Autodesk Inventor part; units mm, degrees
note: some values were not read from the file. Chosen so that the rebuilt part matches the saved one: direction of "Hole2".
(part 17 of 20)
  spline S21 degree 3 poles (10.251041, -15.718972) (10.254521, -15.717406) (10.261436, -15.714294) (10.271248, -15.708633) (10.280531, -15.702321) (10.289255, -15.69531) (10.297429, -15.687643) (10.305055, -15.67934) (10.312135, -15.670426) (10.318671, -15.660926) (10.324667, -15.650864) (10.330124, -15.640264) (10.335046, -15.629149) (10.339434, -15.617543) (10.343295, -15.60547) (10.346618, -15.592951) (10.349454, -15.580017) (10.350882, -15.571212) (10.351603, -15.566761) knots 0 0 0 0 0.05994656 0.11908522 0.17773662 0.23620436 0.29477068 0.35369309 0.41320222 0.47350071 0.53476324 0.59713734 0.66074485 0.72568383 0.79203056 0.85984183 0.92915698 1 1 1 1
  spline S22 degree 3 poles (10.394464, -13.870855) (10.393753, -13.864449) (10.392339, -13.85171) (10.388608, -13.832946) (10.383772, -13.814677) (10.377767, -13.796992) (10.370674, -13.77997) (10.362536, -13.763688) (10.353405, -13.748228) (10.343332, -13.733667) (10.332368, -13.720087) (10.320561, -13.707566) (10.307963, -13.696185) (10.294622, -13.686026) (10.280589, -13.67716) (10.265906, -13.669709) (10.250656, -13.663607) (10.240086, -13.660872) (10.234799, -13.659503) knots 0 0 0 0 0.06847843 0.13617931 0.20309758 0.26921597 0.33450964 0.39895103 0.46251501 0.52518448 0.58695626 0.64784755 0.70790276 0.76720073 0.82586204 0.88405611 0.94200741 1 1 1 1
  spline S23 degree 3 poles (10.107926, -13.682173) (10.104443, -13.684357) (10.097461, -13.688736) (10.087483, -13.696098) (10.077865, -13.704012) (10.068661, -13.712508) (10.059877, -13.721535) (10.051535, -13.731067) (10.04365, -13.74107) (10.036241, -13.751512) (10.029325, -13.762362) (10.02292, -13.773586) (10.017043, -13.785153) (10.011713, -13.797031) (10.006943, -13.809187) (10.002766, -13.821592) (9.999143, -13.834203) (9.997254, -13.842749) (9.996309, -13.847025) knots 0 0 0 0 0.06025982 0.1207868 0.18162334 0.24279657 0.30432017 0.36619627 0.42841724 0.49096745 0.55382495 0.61696316 0.68035239 0.74396143 0.807759 0.87171523 0.93580312 1 1 1 1
  spline S24 degree 3 poles (9.969145, -13.839329) (9.970247, -13.835052) (9.972452, -13.826495) (9.976833, -13.813959) (9.981951, -13.801679) (9.987849, -13.789698) (9.994469, -13.778034) (10.00178, -13.766711) (10.009745, -13.755754) (10.018327, -13.745185) (10.02749, -13.735028) (10.037197, -13.725307) (10.047413, -13.716045) (10.058102, -13.707266) (10.069226, -13.698991) (10.080755, -13.691258) (10.092627, -13.684036) (10.100817, -13.679712) (10.104911, -13.67755) knots 0 0 0 0 0.06083705 0.12173396 0.18278727 0.24406937 0.30563053 0.36750102 0.4296934 0.49220474 0.55501884 0.61810841 0.68143706 0.74496132 0.80863248 0.87239845 0.9362055 1 1 1 1
  spline S25 degree 3 poles (10.204798, -13.648708) (10.21248, -13.648337) (10.227818, -13.647596) (10.250813, -13.649485) (10.273431, -13.653725) (10.295196, -13.660514) (10.315673, -13.669597) (10.334566, -13.680747) (10.351855, -13.693772) (10.367546, -13.708501) (10.381648, -13.724759) (10.394172, -13.742377) (10.405127, -13.761187) (10.414522, -13.781022) (10.422373, -13.801717) (10.428654, -13.823111) (10.433508, -13.845024) (10.43545, -13.859888) (10.436423, -13.867336) knots 0 0 0 0 0.06491361 0.12961858 0.19438015 0.25897481 0.32176837 0.38321901 0.44389655 0.50426715 0.56468953 0.62541836 0.68661292 0.74834873 0.81063045 0.87340478 0.93657257 1 1 1 1
  spline S26 degree 3 poles (10.43359, -13.979425) (10.432261, -13.986039) (10.429641, -13.999072) (10.423361, -14.017768) (10.415518, -14.035336) (10.406031, -14.051702) (10.395025, -14.066825) (10.382574, -14.080659) (10.368764, -14.093159) (10.353678, -14.104281) (10.3374, -14.11398) (10.320012, -14.122213) (10.301596, -14.128938) (10.282235, -14.134109) (10.26201, -14.137691) (10.241006, -14.139605) (10.219289, -14.139949) (10.204661, -14.138753) (10.197237, -14.138147) knots 0 0 0 0 0.06410082 0.12632292 0.18708858 0.24680768 0.30587245 0.36465307 0.42349429 0.48271369 0.54260125 0.60342049 0.66541057 0.72878933 0.79375677 0.86049868 0.92919035 1 1 1 1
  spline S27 degree 3 poles (10.093193, -14.108378) (10.089107, -14.106267) (10.080978, -14.102065) (10.069261, -14.095034) (10.058006, -14.08753) (10.047263, -14.079516) (10.037047, -14.071024) (10.027384, -14.062069) (10.018295, -14.05267) (10.009804, -14.042842) (10.001934, -14.032605) (9.994709, -14.021976) (9.98815, -14.010972) (9.982283, -13.999612) (9.977125, -13.987913) (9.97272, -13.975891) (9.969016, -13.963576) (9.967222, -13.95518) (9.966323, -13.950969) knots 0 0 0 0 0.0658533 0.13104018 0.19559045 0.25953687 0.32291608 0.38576964 0.44814503 0.51009667 0.5716869 0.63298697 0.69407787 0.75505117 0.81600962 0.87706766 0.93835167 1 1 1 1
  spline S28 degree 3 poles (9.993487, -13.958665) (9.994099, -13.962121) (9.995316, -13.969003) (9.997819, -13.979144) (10.000785, -13.989075) (10.004244, -13.998779) (10.008165, -14.008251) (10.01398, -14.020541) (10.022327, -14.035305) (10.033912, -14.051985) (10.046929, -14.06752) (10.061141, -14.081965) (10.071548, -14.090547) (10.07675, -14.094836) knots 0 0 0 0 0.0644506 0.12832403 0.1917227 0.2547379 0.31744987 0.37992792 0.50437187 0.62845768 0.75238919 0.87624484 1 1 1 1
  spline S29 degree 3 poles (10.291069, -14.135155) (10.294549, -14.133589) (10.301464, -14.130478) (10.311276, -14.124817) (10.320559, -14.118505) (10.329282, -14.111493) (10.337457, -14.103826) (10.345083, -14.095523) (10.352163, -14.08661) (10.358699, -14.07711) (10.364695, -14.067048) (10.370152, -14.056448) (10.375074, -14.045333) (10.379462, -14.033727) (10.383323, -14.021653) (10.386646, -14.009135) (10.389482, -13.996201) (10.390909, -13.987395) (10.391631, -13.982945) knots 0 0 0 0 0.05994656 0.11908522 0.17773662 0.23620436 0.29477068 0.35369309 0.41320222 0.47350071 0.53476324 0.59713734 0.66074485 0.72568383 0.79203056 0.85984183 0.92915698 1 1 1 1
  ellipse E534 centre (10.262718, -15.469726) end of major axis (10.283615, -15.718851) minor radius 0.13482 (10.393562, -15.563241) -> (10.396395, -15.451152) ccw
  ellipse E535 centre (10.220759, -15.473246) end of major axis (10.199862, -15.224121) minor radius 0.13482 (10.351603, -15.566761) -> (10.354436, -15.454672) ccw
  ellipse E536 centre (10.302746, -13.88591) end of major axis (10.323643, -14.135035) minor radius 0.13482 (10.43359, -13.979425) -> (10.436423, -13.867336) ccw
  ellipse E537 centre (10.260787, -13.88943) end of major axis (10.23989, -13.640305) minor radius 0.13482 (10.391631, -13.982945) -> (10.394464, -13.870855) ccw
  ellipse E538 centre (10.15921, -15.469521) end of major axis (10.091066, -15.710054) minor radius 0.20633 (9.956281, -15.430841) -> (9.953459, -15.542481) ccw
  ellipse E539 centre (10.199238, -13.885705) end of major axis (10.131093, -14.126238) minor radius 0.20633 (9.996309, -13.847025) -> (9.993487, -13.958665) ccw
  ellipse E540 centre (10.105034, -15.780339) end of major axis (10.392942, -15.787616) minor radius 0.048213 (10.122155, -15.732617) -> (9.948568, -15.736011) ccw
  ellipse E541 centre (10.105034, -15.780339) end of major axis (10.392942, -15.787616) minor radius 0.048213 (10.346718, -15.760066) -> (10.21907, -15.738857) ccw
  ellipse E542 centre (10.105034, -15.780339) end of major axis (9.767142, -15.7718) minor radius 0.056583 (10.388677, -15.756547) -> (10.178195, -15.726878) ccw
  ellipse E543 centre (10.105034, -15.780339) end of major axis (9.767142, -15.7718) minor radius 0.056583 (10.049829, -15.723143) -> (9.921404, -15.728316) ccw
  ellipse E544 centre (10.157666, -13.697823) end of major axis (9.819774, -13.689283) minor radius 0.056583 (10.441308, -13.67403) -> (10.178127, -13.641828) ccw
  ellipse E545 centre (10.157666, -13.697823) end of major axis (9.819774, -13.689283) minor radius 0.056583 (10.040305, -13.641863) -> (9.974036, -13.645799) ccw
  line L655 (10.600693, -15.816612) -> (10.388677, -15.756547)
  line L656 (10.441308, -13.67403) -> (10.472054, -13.682741)
  line L657 (10.560094, -13.707683) -> (10.657791, -13.735361)
  line L658 (10.536886, -15.813942) -> (10.346718, -15.760066)
  line L659 (-10.742088, -15.414015) -> (-10.416365, -15.271775)
  line L660 (-10.379438, -15.155218) -> (-10.439459, -13.966215)
  line L661 (-10.486307, -13.886242) -> (-10.861038, -14.049883)
  ellipse E546 centre (-10.873439, -13.804222) end of major axis (-10.881911, -14.054078) minor radius 0.10517 (-10.971777, -13.909644) -> (-10.861038, -14.049883) ccw
  line L662 (-10.394125, -13.967752) -> (-10.334103, -15.156755)
  line L663 (-10.37103, -15.273312) -> (-10.697321, -15.4158)
  line L664 (-10.975776, -13.750464) -> (-10.972773, -13.750566)
  ellipse E547 centre (-10.421325, -15.17351) end of major axis (-10.424714, -15.273453) minor radius 0.042068 (-10.416365, -15.271775) -> (-10.379438, -15.155218) ccw
  ellipse E548 centre (-10.481347, -13.984507) end of major axis (-10.477958, -13.884564) minor radius 0.042068 (-10.439459, -13.966215) -> (-10.486307, -13.886242) ccw
  ellipse E549 centre (-10.375991, -15.175047) end of major axis (-10.37938, -15.27499) minor radius 0.042068 (-10.37103, -15.273312) -> (-10.334103, -15.156755) ccw
  ellipse E550 centre (-10.436013, -13.986044) end of major axis (-10.432624, -13.886102) minor radius 0.042068 (-10.394125, -13.967752) -> (-10.432624, -13.886102) ccw
  line L665 (-10.477958, -13.884564) -> (-10.432624, -13.886102)
  ellipse E551 centre (9.593076, -13.995154) end of major axis (9.580639, -13.895931) minor radius 0.05049 (9.606839, -13.905631) -> (9.581879, -13.895806) ccw
  line L666 (9.581879, -13.895806) -> (9.525543, -13.900087)
  line L667 (10.228683, -15.760397) -> (10.072847, -15.769343)
  line L668 (10.1976, -15.772588) -> (10.25938, -15.769041)
  ellipse E552 centre (10.515718, -15.496033) end of major axis (10.598446, -15.260117) minor radius 0.210338 (10.301924, -15.548655) -> (10.303804, -15.563691) ccw
  ellipse E553 centre (10.515718, -15.496033) end of major axis (10.598446, -15.260117) minor radius 0.210338 (10.30944, -15.452383) -> (10.303787, -15.480748) ccw
  ellipse E554 centre (10.595673, -13.916931) end of major axis (10.678401, -13.681016) minor radius 0.210338 (10.389395, -13.873281) -> (10.383759, -13.984589) ccw
  spline S30 degree 3 poles (10.639222, -15.311893) (10.635884, -15.309378) (10.629234, -15.304367) (10.618664, -15.297765) (10.607739, -15.291925) (10.59643, -15.286944) (10.584771, -15.282844) (10.572777, -15.279666) (10.56047, -15.277447) (10.54787, -15.276224) (10.534997, -15.276034) (10.521873, -15.276915) (10.50855, -15.278899) (10.495208, -15.281972) (10.482035, -15.286085) (10.469204, -15.291185) (10.456712, -15.297151) (10.448757, -15.301841) (10.444771, -15.30419) knots 0 0 0 0 0.06027236 0.12008459 0.17956335 0.23886314 0.2981675 0.35768957 0.41767151 0.47838294 0.54011829 0.60319317 0.66794006 0.7342313 0.80052522 0.86682566 0.93327954 1 1 1 1
  spline S31 degree 3 poles (10.349743, -15.416894) (10.348235, -15.42049) (10.345216, -15.427688) (10.341299, -15.438734) (10.337796, -15.449935) (10.335894, -15.457528) (10.334942, -15.461326) knots 0 0 0 0 0.24945299 0.49932153 0.74952532 1 1 1 1
  spline S32 degree 3 poles (10.30944, -15.452383) (10.310327, -15.449265) (10.312103, -15.443026) (10.315351, -15.433844) (10.319008, -15.424803) (10.323103, -15.415925) (10.327606, -15.407214) (10.332514, -15.398686) (10.33778, -15.390328) (10.341586, -15.38494) (10.343493, -15.38224) knots 0 0 0 0 0.12403661 0.24815991 0.37248981 0.49712476 0.62214288 0.74760322 0.87354721 1 1 1 1
  spline S33 degree 3 poles (10.420747, -15.311069) (10.425243, -15.308365) (10.434233, -15.302957) (10.448239, -15.295782) (10.462562, -15.289332) (10.477187, -15.283704) (10.492051, -15.278915) (10.5071, -15.275003) (10.52228, -15.271999) (10.537537, -15.269939) (10.552815, -15.268854) (10.56806, -15.26878) (10.583218, -15.26975) (10.598233, -15.2718) (10.613053, -15.274957) (10.627529, -15.279263) (10.641528, -15.28456) (10.650393, -15.288965) (10.654779, -15.291144) knots 0 0 0 0 0.06405989 0.1281006 0.19204727 0.25582983 0.3193861 0.38266496 0.44562961 0.50826114 0.57056212 0.63256041 0.69431295 0.75590946 0.81747579 0.87917562 0.94021367 1 1 1 1
  spline S34 degree 3 poles (10.642411, -15.748997) (10.637993, -15.750336) (10.629077, -15.753038) (10.615271, -15.756008) (10.601047, -15.758216) (10.586405, -15.759564) (10.57138, -15.760062) (10.555998, -15.759689) (10.540286, -15.758432) (10.524272, -15.756276) (10.50799, -15.753204) (10.491611, -15.749258) (10.475393, -15.744428) (10.459591, -15.73876) (10.4443, -15.73231) (10.429573, -15.725088) (10.415399, -15.717193) (10.406416, -15.711291) (10.401949, -15.708356) knots 0 0 0 0 0.0549764 0.11096338 0.16806833 0.22639244 0.28603139 0.34707614 0.40961367 0.47372767 0.53949927 0.6069434 0.67436537 0.7409998 0.80686402 0.87197412 0.93634658 1 1 1 1
  spline S35 degree 3 poles (10.333198, -15.638612) (10.331414, -15.635736) (10.32785, -15.629994) (10.323033, -15.621083) (10.31863, -15.611983) (10.31469, -15.602682) (10.311213, -15.593194) (10.308225, -15.583524) (10.305691, -15.57369) (10.304434, -15.567029) (10.303804, -15.563691) knots 0 0 0 0 0.12529925 0.25024005 0.37494166 0.49953681 0.62417216 0.7490086 0.87422136 1 1 1 1
  spline S36 degree 3 poles (10.329306, -15.572633) (10.329595, -15.574574) (10.33017, -15.578445) (10.331249, -15.584202) (10.332481, -15.589901) (10.333878, -15.595536) (10.335431, -15.601108) (10.337142, -15.606614) (10.338994, -15.612058) (10.340356, -15.615636) (10.341036, -15.617422) knots 0 0 0 0 0.12682999 0.25300914 0.37860655 0.50368723 0.62831214 0.75253809 0.87641783 1 1 1 1
  spline S37 degree 3 poles (10.623456, -15.757558) (10.625199, -15.756839) (10.62867, -15.755407) (10.633738, -15.752997) (10.638684, -15.750427) (10.641874, -15.748549) (10.643465, -15.747612) knots 0 0 0 0 0.25282857 0.50351543 0.75244628 1 1 1 1
  spline S38 degree 3 poles (10.654391, -13.701114) (10.651269, -13.700442) (10.645002, -13.699093) (10.635416, -13.697812) (10.625672, -13.697086) (10.615766, -13.696986) (10.605712, -13.697514) (10.595517, -13.698691) (10.585226, -13.700526) (10.574945, -13.703003) (10.564785, -13.706095) (10.554824, -13.709766) (10.545074, -13.713995) (10.535551, -13.718761) (10.526263, -13.724041) (10.517233, -13.729824) (10.508444, -13.736052) (10.502841, -13.740567) (10.500032, -13.742829) knots 0 0 0 0 0.05778221 0.11602992 0.17490487 0.23457915 0.29523385 0.35705764 0.42024514 0.48436692 0.54838884 0.61238964 0.67645987 0.74067474 0.80509501 0.86976792 0.93472837 1 1 1 1
  spline S39 degree 3 poles (10.389395, -13.873281) (10.3897, -13.872169) (10.390311, -13.869944) (10.391303, -13.866627) (10.392345, -13.863326) (10.393089, -13.861141) (10.393462, -13.860049) knots 0 0 0 0 0.24996578 0.49993063 0.74993068 1 1 1 1
  spline S40 degree 3 poles (10.475835, -13.749315) (10.482485, -13.744399) (10.495798, -13.734557) (10.517269, -13.722015) (10.539622, -13.711219) (10.562762, -13.702453) (10.586446, -13.695807) (10.606512, -13.692148) (10.62262, -13.690422) (10.634679, -13.689759) (10.646716, -13.68968) (10.654706, -13.69018) (10.658695, -13.69043) knots 0 0 0 0 0.12626187 0.25278671 0.37919835 0.50514032 0.63031299 0.75451273 0.81623998 0.87771389 0.93895544 1 1 1 1
  spline S41 degree 3 poles (10.656162, -14.18075) (10.647734, -14.180716) (10.634964, -14.180664) (10.617843, -14.179005) (10.604672, -14.177201) (10.591315, -14.174763) (10.573319, -14.170701) (10.55117, -14.164202) (10.525666, -14.154126) (10.501636, -14.142007) (10.48292, -14.130222) (10.468841, -14.119935) (10.462196, -14.114415) (10.458888, -14.111667) knots 0 0 0 0 0.11836757 0.17935651 0.24161124 0.30518476 0.370129 0.50087366 0.62916185 0.75504201 0.87860366 0.93956774 1 1 1 1
  spline S42 degree 3 poles (10.388048, -14.003652) (10.387624, -14.002085) (10.386776, -13.998946) (10.385653, -13.994195) (10.38463, -13.989411) (10.38405, -13.986198) (10.383759, -13.984589) knots 0 0 0 0 0.24922132 0.49890182 0.74913063 1 1 1 1
  ellipse E555 centre (10.54122, -15.504976) end of major axis (10.458492, -15.740891) minor radius 0.210338 (10.334942, -15.461326) -> (10.32839, -15.49627) ccw
  ellipse E556 centre (10.54122, -15.504976) end of major axis (10.458492, -15.740891) minor radius 0.210338 (10.326884, -15.551145) -> (10.329306, -15.572633) ccw
  ellipse E557 centre (10.466428, -15.817098) end of major axis (10.754059, -15.831661) minor radius 0.051474 (10.360563, -15.763989) -> (10.321007, -15.765504) ccw
  ellipse E558 centre (10.466428, -15.817098) end of major axis (10.754059, -15.831661) minor radius 0.051474 (10.641488, -15.784784) -> (10.427949, -15.764137) ccw
  ellipse E559 centre (10.466428, -15.817098) end of major axis (10.12886, -15.800006) minor radius 0.06041 (10.647208, -15.774877) -> (10.39844, -15.75452) ccw
  ellipse E560 centre (10.466428, -15.817098) end of major axis (10.12886, -15.800006) minor radius 0.06041 (10.327397, -15.755166) -> (10.296227, -15.756521) ccw
  ellipse E561 centre (10.571558, -13.74078) end of major axis (10.233991, -13.723688) minor radius 0.06041 (10.657553, -13.686505) -> (10.45631, -13.67828) ccw
  line L669 (11.644785, -15.760338) -> (11.949094, -15.867049)
  line L670 (12.005073, -15.786671) -> (12.065276, -14.597677)
  line L671 (12.019247, -14.481528) -> (11.714938, -14.374816)
  line L672 (11.906158, -15.869514) -> (11.643913, -15.777553)
  ellipse E562 centre (11.954069, -15.768785) end of major axis (11.959801, -15.868621) minor radius 0.051008 (11.949094, -15.867049) -> (12.005073, -15.786671) ccw
  ellipse E563 centre (12.014272, -14.579791) end of major axis (12.00854, -14.479956) minor radius 0.051008 (12.065276, -14.597677) -> (12.019247, -14.481528) ccw
  ellipse E564 centre (11.911134, -15.77125) end of major axis (11.916865, -15.871086) minor radius 0.051008 (11.906158, -15.869514) -> (11.916865, -15.871086) ccw
  line L673 (11.959801, -15.868621) -> (11.916865, -15.871086)
  line L674 (-10.282197, -15.750913) -> (-10.32851, -15.76587)
  line L675 (-10.462033, -13.717932) -> (-10.295788, -13.664245)
  line L676 (-10.237418, -15.754127) -> (-10.280706, -15.768106)
  line L677 (-10.282197, -15.750913) -> (-10.28285, -15.650678)
  ellipse E565 centre (-10.171636, -15.614763) end of major axis (-10.153742, -15.365405) minor radius 0.110059 (-10.173244, -15.367879) -> (-10.28285, -15.650678) ccw
  line L678 (-10.173244, -15.367879) -> (-9.775271, -15.239359)
  line L679 (-9.731428, -15.126239) -> (-9.739211, -13.931318)
  line L680 (-9.78434, -13.84693) -> (-10.086187, -13.944408)
  ellipse E566 centre (-10.183921, -13.728565) end of major axis (-10.166027, -13.479207) minor radius 0.110059 (-10.295135, -13.76448) -> (-10.27236, -13.904301) ccw
  line L681 (-10.295135, -13.76448) -> (-10.295788, -13.664245)
  line L682 (-9.694432, -13.934531) -> (-9.686649, -15.129453)
  line L683 (-10.251009, -13.667459) -> (-10.250356, -13.767694)
  ellipse E567 centre (-10.139142, -13.731779) end of major axis (-10.157036, -13.981138) minor radius 0.110059 (-10.250356, -13.767694) -> (-10.234077, -13.888278) ccw
  line L684 (-9.730492, -15.242572) -> (-10.128465, -15.371092)
  ellipse E568 centre (-10.126857, -15.617977) end of major axis (-10.108963, -15.368618) minor radius 0.110059 (-10.128465, -15.371092) -> (-10.238071, -15.653892) ccw
  line L685 (-10.238071, -15.653892) -> (-10.237418, -15.754127)
  line L686 (-10.295788, -13.664245) -> (-10.251009, -13.667459)
  line L687 (-10.237418, -15.754127) -> (-10.282197, -15.750913)
  ellipse E569 centre (-9.775914, -15.140605) end of major axis (-9.783071, -15.240349) minor radius 0.044024 (-9.775271, -15.239359) -> (-9.731428, -15.126239) ccw
  ellipse E570 centre (-9.783697, -13.945684) end of major axis (-9.776539, -13.845941) minor radius 0.044024 (-9.739211, -13.931318) -> (-9.78434, -13.84693) ccw
  ellipse E571 centre (-9.731135, -15.143819) end of major axis (-9.738292, -15.243562) minor radius 0.044024 (-9.730492, -15.242572) -> (-9.686649, -15.129453) ccw
  ellipse E572 centre (-9.738918, -13.948897) end of major axis (-9.73176, -13.849154) minor radius 0.044024 (-9.694432, -13.934531) -> (-9.73176, -13.849154) ccw
  line L688 (-9.776539, -13.845941) -> (-9.73176, -13.849154)
  line L689 (9.741809, -15.714548) -> (9.713889, -15.716876)
  line L690 (9.755718, -13.627882) -> (9.54778, -13.645222)
  line L691 (9.717209, -15.725656) -> (9.766621, -15.721535)
  ellipse E573 centre (9.954871, -15.447073) end of major axis (10.022637, -15.206433) minor radius 0.214215 (9.743847, -15.40877) -> (9.743102, -15.520632) ccw
  ellipse E574 centre (9.965449, -13.860101) end of major axis (10.033215, -13.619461) minor radius 0.214215 (9.754425, -13.821798) -> (9.75368, -13.93366) ccw
  spline S43 degree 3 poles (10.161609, -15.43493) (10.159715, -15.421319) (10.155981, -15.394491) (10.143629, -15.356301) (10.126915, -15.321298) (10.105779, -15.290275) (10.080734, -15.263978) (10.052132, -15.243202) (10.02562, -15.231202) (10.003342, -15.225299) (9.986022, -15.222758) (9.968175, -15.222215) (9.949862, -15.223769) (9.931292, -15.227486) (9.912861, -15.233296) (9.894979, -15.241075) (9.872148, -15.253851) (9.845774, -15.274045) (9.818449, -15.303667) (9.79601, -15.337809) (9.778457, -15.375371) (9.771933, -15.402262) (9.76866, -15.415757) knots 0 0 0 0 0.06705351 0.13217076 0.19521445 0.25608707 0.314845 0.37183317 0.42783149 0.45589727 0.48426542 0.51319288 0.54296576 0.57389196 0.60556318 0.63723227 0.66902668 0.73324746 0.79861392 0.865047 0.93227307 1 1 1 1
  spline S44 degree 3 poles (9.743847, -15.40877) (9.74561, -15.401972) (9.749142, -15.388353) (9.759841, -15.362104) (9.777917, -15.331047) (9.806113, -15.29784) (9.839536, -15.269137) (9.877046, -15.245654) (9.917484, -15.228106) (9.959703, -15.217251) (9.995597, -15.214449) (10.023891, -15.216419) (10.044692, -15.220067) (10.064729, -15.225906) (10.083644, -15.233775) (10.101176, -15.243484) (10.122621, -15.258624) (10.146205, -15.281633) (10.168957, -15.314274) (10.186276, -15.350802) (10.198786, -15.390122) (10.202929, -15.417508) (10.205017, -15.431311) knots 0 0 0 0 0.03133748 0.06278121 0.12629735 0.19093644 0.25645898 0.32231967 0.3878749 0.45257734 0.51618281 0.54767829 0.57907039 0.61032535 0.64070557 0.67038635 0.69964994 0.75776174 0.81647804 0.87644136 0.93772561 1 1 1 1
  spline S45 degree 3 poles (10.204269, -15.543623) (10.201908, -15.556082) (10.19731, -15.580347) (10.182423, -15.613721) (10.162365, -15.642715) (10.137107, -15.666876) (10.107303, -15.685863) (10.073437, -15.699346) (10.036019, -15.707019) (9.995527, -15.70858) (9.952917, -15.70378) (9.910141, -15.692921) (9.869514, -15.675879) (9.832831, -15.653493) (9.8009, -15.626287) (9.778813, -15.599883) (9.764423, -15.576962) (9.755396, -15.558956) (9.748021, -15.540185) (9.744744, -15.52716) (9.743102, -15.520632) knots 0 0 0 0 0.06022667 0.11730293 0.17254203 0.22724068 0.28263107 0.33984452 0.39989686 0.46369518 0.53205848 0.6034638 0.67318901 0.7411164 0.8073508 0.87214279 0.90417982 0.93607992 0.96796844 1 1 1 1
  spline S46 degree 3 poles (9.767914, -15.52762) (9.768579, -15.530918) (9.769903, -15.537491) (9.772511, -15.547175) (9.775543, -15.556665) (9.780179, -15.569018) (9.787041, -15.583954) (9.796859, -15.600989) (9.808104, -15.617064) (9.820661, -15.632099) (9.83431, -15.646148) (9.844267, -15.654569) (9.849243, -15.658778) knots 0 0 0 0 0.06406043 0.12763921 0.19082759 0.25370622 0.37876994 0.50330734 0.62760512 0.75181377 0.87596664 1 1 1 1
  spline S47 degree 3 poles (10.062691, -15.704262) (10.066245, -15.702726) (10.073294, -15.699681) (10.083257, -15.694021) (10.092625, -15.687651) (10.101369, -15.68052) (10.109507, -15.672678) (10.117042, -15.664148) (10.123983, -15.65496) (10.130337, -15.64514) (10.136112, -15.634717) (10.141316, -15.623719) (10.145956, -15.612172) (10.15004, -15.600103) (10.153578, -15.587539) (10.156565, -15.574507) (10.159056, -15.561037) (10.160254, -15.551877) (10.160861, -15.547243) knots 0 0 0 0 0.05963345 0.11825449 0.17626219 0.23403402 0.29191894 0.35023204 0.40925111 0.46921525 0.53032509 0.59274441 0.65660269 0.7219981 0.78900076 0.85765603 0.92798753 1 1 1 1
  spline S48 degree 3 poles (10.172187, -13.847958) (10.170293, -13.834347) (10.166559, -13.807519) (10.154207, -13.769329) (10.137493, -13.734326) (10.116357, -13.703303) (10.091312, -13.677006) (10.06271, -13.65623) (10.036198, -13.64423) (10.01392, -13.638327) (9.9966, -13.635786) (9.978753, -13.635243) (9.96044, -13.636796) (9.94187, -13.640514) (9.923439, -13.646324) (9.905556, -13.654102) (9.882726, -13.666879) (9.856351, -13.687073) (9.829027, -13.716695) (9.806588, -13.750837) (9.789035, -13.788399) (9.782511, -13.81529) (9.779238, -13.828785) knots 0 0 0 0 0.06705351 0.13217076 0.19521445 0.25608707 0.314845 0.37183317 0.42783149 0.45589727 0.48426542 0.51319288 0.54296576 0.57389196 0.60556318 0.63723227 0.66902668 0.73324746 0.79861392 0.865047 0.93227307 1 1 1 1
  spline S49 degree 3 poles (9.754425, -13.821798) (9.756188, -13.815) (9.75972, -13.80138) (9.770419, -13.775132) (9.788495, -13.744075) (9.816691, -13.710868) (9.850113, -13.682165) (9.887624, -13.658681) (9.928062, -13.641134) (9.97028, -13.630278) (10.006175, -13.627477) (10.034469, -13.629447) (10.05527, -13.633095) (10.075307, -13.638934) (10.094222, -13.646803) (10.111754, -13.656512) (10.133199, -13.671652) (10.156783, -13.69466) (10.179535, -13.727301) (10.196854, -13.76383) (10.209364, -13.80315) (10.213507, -13.830536) (10.215595, -13.844338) knots 0 0 0 0 0.03133748 0.06278121 0.12629735 0.19093644 0.25645898 0.32231967 0.3878749 0.45257734 0.51618281 0.54767829 0.57907039 0.61032535 0.64070557 0.67038635 0.69964994 0.75776174 0.81647804 0.87644136 0.93772561 1 1 1 1
  spline S50 degree 3 poles (10.214846, -13.956651) (10.212486, -13.969109) (10.207887, -13.993374) (10.193001, -14.026749) (10.172943, -14.055743) (10.147685, -14.079904) (10.117881, -14.098891) (10.084015, -14.112373) (10.046597, -14.120047) (10.006105, -14.121608) (9.963495, -14.116808) (9.920719, -14.105949) (9.880092, -14.088907) (9.843409, -14.06652) (9.811478, -14.039315) (9.78939, -14.012911) (9.775001, -13.98999) (9.765974, -13.971984) (9.758599, -13.953213) (9.755322, -13.940187) (9.75368, -13.93366) knots 0 0 0 0 0.06022667 0.11730293 0.17254203 0.22724068 0.28263107 0.33984452 0.39989686 0.46369518 0.53205848 0.6034638 0.67318901 0.7411164 0.8073508 0.87214279 0.90417982 0.93607992 0.96796844 1 1 1 1
  spline S51 degree 3 poles (9.778492, -13.940648) (9.779157, -13.943946) (9.780481, -13.950519) (9.783089, -13.960202) (9.786121, -13.969693) (9.790757, -13.982045) (9.797618, -13.996982) (9.807437, -14.014017) (9.818682, -14.030092) (9.831238, -14.045127) (9.844888, -14.059176) (9.854845, -14.067597) (9.859821, -14.071806) knots 0 0 0 0 0.06406043 0.12763921 0.19082759 0.25370622 0.37876994 0.50330734 0.62760512 0.75181377 0.87596664 1 1 1 1
  spline S52 degree 3 poles (10.073269, -14.117289) (10.076823, -14.115754) (10.083872, -14.112709) (10.093835, -14.107048) (10.103202, -14.100679) (10.111947, -14.093548) (10.120085, -14.085706) (10.12762, -14.077176) (10.134561, -14.067987) (10.140915, -14.058168) (10.14669, -14.047745) (10.151894, -14.036747) (10.156534, -14.0252) (10.160618, -14.013131) (10.164156, -14.000567) (10.167143, -13.987534) (10.169634, -13.974065) (10.170832, -13.964905) (10.171439, -13.960271) knots 0 0 0 0 0.05963345 0.11825449 0.17626219 0.23403402 0.29191894 0.35023204 0.40925111 0.46921525 0.53032509 0.59274441 0.65660269 0.7219981 0.78900076 0.85765603 0.92798753 1 1 1 1
  ellipse E575 centre (10.083833, -15.453446) end of major axis (10.104608, -15.702581) minor radius 0.122746 (10.204269, -15.543623) -> (10.205017, -15.431311) ccw
  ellipse E576 centre (10.040425, -15.457065) end of major axis (10.01965, -15.20793) minor radius 0.122746 (10.160861, -15.547243) -> (10.161609, -15.43493) ccw
  ellipse E577 centre (10.094411, -13.866473) end of major axis (10.115186, -14.115609) minor radius 0.122746 (10.214846, -13.956651) -> (10.215595, -13.844338) ccw
  ellipse E578 centre (10.051003, -13.870093) end of major axis (10.030228, -13.620958) minor radius 0.122746 (10.171439, -13.960271) -> (10.172187, -13.847958) ccw
  ellipse E579 centre (9.979683, -15.454061) end of major axis (9.911916, -15.694701) minor radius 0.214215 (9.76866, -15.415757) -> (9.767914, -15.52762) ccw
  ellipse E580 centre (9.990261, -13.867088) end of major axis (9.922494, -14.107729) minor radius 0.214215 (9.779238, -13.828785) -> (9.778492, -13.940648) ccw
  ellipse E581 centre (9.909541, -15.761783) end of major axis (10.197534, -15.763703) minor radius 0.045287 (10.15957, -15.740933) -> (9.766621, -15.721535) ccw
  ellipse E582 centre (9.909541, -15.761783) end of major axis (9.571548, -15.75953) minor radius 0.05315 (10.202977, -15.737314) -> (9.741809, -15.714548) ccw
  ellipse E583 centre (9.923449, -13.675117) end of major axis (9.585457, -13.672864) minor radius 0.05315 (10.216886, -13.650648) -> (9.755718, -13.627882) ccw
  line L692 (10.362182, -15.782147) -> (10.202977, -15.737314)
  line L693 (10.216886, -13.650648) -> (10.233521, -13.655332)
  line L694 (10.249221, -13.659754) -> (10.262113, -13.663384)
  line L695 (10.320149, -15.786154) -> (10.15957, -15.740933)
  line L696 (-10.556192, -13.681536) -> (-10.449696, -13.686518)
  ellipse E584 centre (10.463699, -13.355926) end of major axis (10.3792, -13.654187) minor radius 0.255849 (10.455977, -13.661454) -> (10.469835, -13.659859) ccw
  line L697 (10.469835, -13.659859) -> (10.537125, -13.678923)
  line L698 (10.406363, -13.665615) -> (10.455977, -13.661454)
  arc A6 (-11.816794, -13.823521) -> (-11.715647, -13.93349) centre (-11.544781, -13.674831) ccw
  ellipse E585 centre (10.458723, -13.771809) end of major axis (10.900657, -13.794186) minor radius 0.079087 (10.657954, -13.710891) -> (10.64589, -13.709249) ccw
  arc A7 (11.737457, -13.930058) -> (11.862789, -13.807718) centre (11.592403, -13.656089) ccw
  ellipse E586 centre (-10.265604, -13.334113) end of major axis (-10.170338, -13.629112) minor radius 0.274042 (-10.278389, -13.638755) -> (-10.26361, -13.64025) ccw
  line L699 (-10.293774, -13.643724) -> (-10.278389, -13.638755)
  line L700 (-10.26361, -13.64025) -> (-10.124104, -13.650261)
  ellipse E587 centre (9.661276, -13.302469) end of major axis (9.687037, -13.611397) minor radius 0.152204 (9.650555, -13.605672) -> (9.659236, -13.608606) ccw
  line L701 (9.550807, -13.61399) -> (9.650555, -13.605672)
  ellipse E588 centre (10.224961, -13.330181) end of major axis (10.14093, -13.628574) minor radius 0.265627 (10.22292, -13.636317) -> (10.237248, -13.634689) ccw
  line L702 (10.237248, -13.634689) -> (10.287053, -13.648714)
  line L703 (10.17142, -13.640612) -> (10.22292, -13.636317)
  line L704 (9.659236, -13.608606) -> (9.711987, -13.623461)
  ellipse E589 centre (9.802019, -13.701571) end of major axis (10.24451, -13.70452) minor radius 0.069582 (10.022187, -13.642643) -> (9.996076, -13.640297) ccw
  arc A8 (-10.355944, -15.764586) -> (-10.490112, -15.788282) centre (-10.370431, -16.074248) ccw
  line L705 (-10.490112, -15.788282) -> (-10.535858, -15.807427)
  line L706 (-10.030129, -15.779829) -> (-10.355944, -15.764586)
  arc A9 (-10.762476, -15.815509) -> (-10.777672, -15.821671) centre (-10.653611, -16.105765) ccw
  arc A10 (-10.643105, -15.795943) -> (-10.734549, -15.806517) centre (-10.653611, -16.105765) ccw
  line L707 (-10.777672, -15.821671) -> (-10.867854, -15.861053)
  line L708 (-10.518512, -15.800167) -> (-10.643105, -15.795943)
  arc A11 (-9.397515, -21.165082) -> (-9.395444, -21.164343) centre (-9.799927, -20.034567) ccw
  line L709 (9.186636, -20.230589) -> (9.285399, -21.174429)
  line L710 (-9.178745, -20.229192) -> (-9.277652, -21.173018)
  arc A12 (9.403193, -21.165772) -> (9.405264, -21.166512) centre (9.807848, -20.036058) ccw
  arc A13 (6.406707, -24.006558) -> (6.522311, -23.980999) centre (6.20577, -22.823501) ccw
  line L711 (6.709268, -22.715225) -> (6.722153, -22.773503)
  arc A14 (-6.51499, -23.980007) -> (-6.399391, -24.005584) centre (-6.198273, -22.822558) ccw
  line L712 (-6.701755, -22.714205) -> (-6.714649, -22.772482)
  arc A15 (-10.26245, -22.988371) -> (-9.772476, -23.022679) centre (-9.93542, -21.833793) ccw
  line L713 (-11.030091, -10.363726) -> (-11.020632, -10.551114)
  line L714 (-10.969032, -11.573283) -> (-10.961826, -11.71603)
  line L715 (-10.651662, -17.860261) -> (-10.534824, -20.174762)
  line L716 (-10.480511, -21.25069) -> (-10.446106, -21.932231)
  arc A16 (-7.348548, -23.890588) -> (-7.2302, -23.896817) centre (-7.226379, -22.696823) ccw
  line L717 (-6.711421, -22.711164) -> (-6.714649, -22.772482)
  line L718 (-7.70072, -21.910773) -> (-7.751062, -22.867245)
  line L719 (5.511675, -21.765174) -> (5.527948, -21.84198)
  arc A17 (8.895723, -24.211337) -> (9.194656, -24.177647) centre (8.911858, -23.011445) ccw
  line L720 (9.338337, -22.197066) -> (9.444354, -23.137756)
  line L721 (8.313899, -22.304271) -> (8.420834, -23.253108)
  arc A18 (-9.187365, -24.176249) -> (-8.888437, -24.209984) centre (-8.90439, -23.010091) ccw
  line L722 (-8.306323, -22.303007) -> (-8.413402, -23.251828)
  line L723 (-9.330745, -22.195646) -> (-9.436905, -23.13632)
  line L724 (-5.504017, -21.764336) -> (-5.520302, -21.84114)
  arc A19 (7.237534, -23.897917) -> (7.355882, -23.891706) centre (7.233895, -22.697923) ccw
  line L725 (7.708356, -21.911945) -> (7.758552, -22.868424)
  line L726 (6.718935, -22.712185) -> (6.722153, -22.773503)
  arc A20 (9.779942, -23.024166) -> (10.269921, -22.989933) centre (9.943067, -21.835305) ccw
  line L727 (11.039483, -10.365404) -> (11.029995, -10.552791)
  line L728 (10.97824, -11.574952) -> (10.972655, -11.685252)
  line L729 (10.661472, -17.831088) -> (10.542724, -20.176365)
  line L730 (10.488247, -21.252284) -> (10.453738, -21.933821)
  line L731 (-9.181474, -10.421055) -> (-9.181206, -10.462165)
  line L732 (-9.133538, -17.780681) -> (-9.130352, -18.269798)
  line L733 (8.996999, -17.663203) -> (9.146884, -19.198697)
  line L734 (-8.988717, -17.661835) -> (-9.138836, -19.197307)
  line L735 (9.190857, -10.422453) -> (9.190583, -10.463563)
  line L736 (9.141873, -17.771436) -> (9.138542, -18.271187)
  ellipse E590 centre (-10.18616, -4.659564) end of major axis (-11.885624, -4.702256) minor radius 0.28459 (-11.372081, -4.484612) -> (-11.885624, -4.702256) ccw
  line L737 (-11.881763, -4.855925) -> (-11.885624, -4.702256)
  ellipse E591 centre (10.196419, -4.661114) end of major axis (11.895876, -4.704065) minor radius 0.28459 (11.895876, -4.704065) -> (11.382367, -4.486342) ccw
  line L738 (11.891993, -4.857733) -> (11.895876, -4.704065)
  ellipse E592 centre (-10.709252, -6.504497) end of major axis (-12.40709, -6.590205) minor radius 0.303839 (-11.657242, -6.298438) -> (-12.40709, -6.590205) ccw
  line L739 (-12.399854, -6.733536) -> (-12.40709, -6.590205)
  ellipse E593 centre (10.71923, -6.506127) end of major axis (12.417055, -6.592093) minor radius 0.303839 (12.417055, -6.592093) -> (11.667252, -6.300212) ccw
  line L740 (12.409798, -6.735422) -> (12.417055, -6.592093)
  ellipse E594 centre (7.105738, -3.589226) end of major axis (8.797696, -3.424068) minor radius 0.097712 (8.797696, -3.424068) -> (8.280307, -3.404289) ccw
  line L741 (8.822055, -3.673614) -> (8.797696, -3.424068)
  ellipse E595 centre (-7.095315, -3.588146) end of major axis (-8.787248, -3.42273) minor radius 0.097712 (-8.269856, -3.403031) -> (-8.787248, -3.42273) ccw
  line L742 (-8.811645, -3.672273) -> (-8.787248, -3.42273)
  ellipse E596 centre (-10.109408, -7.714853) end of major axis (-8.609881, -7.677184) minor radius 0.251109 (-9.236268, -7.489321) -> (-9.859849, -7.461077) ccw
  ellipse E597 centre (-10.109408, -7.714853) end of major axis (-8.210008, -7.667139) minor radius 0.318071 (-9.228111, -7.411487) -> (-11.173605, -7.477296) ccw
  ellipse E598 centre (-10.178732, -4.955237) end of major axis (-12.078133, -5.002952) minor radius 0.318071 (-10.880624, -4.676726) -> (-12.078133, -5.002952) ccw
  line L743 (-12.043501, -6.381552) -> (-12.078133, -5.002952)
  ellipse E599 centre (7.455781, -8.638064) end of major axis (9.345463, -8.440328) minor radius 0.08119 (9.187291, -8.489909) -> (9.128782, -8.425367) ccw
  ellipse E600 centre (7.164645, -5.855813) end of major axis (9.054328, -5.658076) minor radius 0.08119 (8.943607, -5.642471) -> (8.543101, -5.655998) ccw
  line L744 (9.345463, -8.440328) -> (9.140443, -6.481034)
  ellipse E601 centre (-7.446126, -8.636931) end of major axis (-9.335779, -8.438907) minor radius 0.08119 (-9.119096, -8.42398) -> (-9.177614, -8.488512) ccw
  ellipse E602 centre (-7.154568, -5.854724) end of major axis (-9.04422, -5.656699) minor radius 0.08119 (-8.532993, -5.654699) -> (-8.933496, -5.641111) ccw
  line L745 (-9.335779, -8.438907) -> (-9.13046, -6.479645)
  ellipse E603 centre (10.119203, -7.716391) end of major axis (11.618724, -7.754289) minor radius 0.251109 (9.869682, -7.462577) -> (9.246097, -7.490727) ccw
  ellipse E604 centre (10.119203, -7.716391) end of major axis (12.018597, -7.764395) minor radius 0.318071 (11.183436, -7.478996) -> (9.237952, -7.412891) ccw
  ellipse E605 centre (10.188947, -4.956786) end of major axis (12.08834, -5.00479) minor radius 0.318071 (12.08834, -5.00479) -> (10.89088, -4.678382) ccw
  line L746 (12.053499, -6.383384) -> (12.08834, -5.00479)
  ellipse E606 centre (-10.555477, -9.550703) end of major axis (-12.05357, -9.626328) minor radius 0.268093 (-9.274709, -9.348863) -> (-11.745841, -9.771854) ccw
  ellipse E607 centre (-10.555477, -9.550703) end of major axis (-12.453061, -9.646494) minor radius 0.339584 (-9.262275, -9.238683) -> (-11.740677, -9.874152) ccw
  ellipse E608 centre (-10.69437, -6.799291) end of major axis (-12.591954, -6.895082) minor radius 0.339584 (-11.209708, -6.497247) -> (-12.591954, -6.895082) ccw
  line L747 (-12.453061, -9.646494) -> (-12.591954, -6.895082)
  ellipse E609 centre (7.512272, -10.5929) end of major axis (9.40032, -10.380115) minor radius 0.04047 (9.10107, -10.435925) -> (9.09598, -10.392324) ccw
  ellipse E610 centre (7.198765, -7.811146) end of major axis (9.086812, -7.59836) minor radius 0.04047 (9.037379, -7.594768) -> (8.771321, -7.611459) ccw
  line L748 (9.40032, -10.380115) -> (9.181511, -8.438625)
  ellipse E611 centre (-7.502915, -10.591758) end of major axis (-9.39093, -10.378686) minor radius 0.04047 (-9.086592, -10.390941) -> (-9.091689, -10.434542) ccw
  ellipse E612 centre (-7.188985, -7.810052) end of major axis (-9.077, -7.596979) minor radius 0.04047 (-8.761511, -7.610126) -> (-9.027566, -7.593394) ccw
  line L749 (-9.39093, -10.378686) -> (-9.171826, -8.437229)
  ellipse E613 centre (10.564993, -9.552309) end of major axis (12.063074, -9.628162) minor radius 0.268093 (11.755323, -9.773641) -> (9.284255, -9.350274) ccw
  ellipse E614 centre (10.564993, -9.552309) end of major axis (12.462562, -9.648389) minor radius 0.339584 (11.750144, -9.875938) -> (9.271838, -9.240092) ccw
  ellipse E615 centre (10.704304, -6.800919) end of major axis (12.601873, -6.896998) minor radius 0.339584 (12.601873, -6.896998) -> (11.219688, -6.498953) ccw
  line L750 (12.462562, -9.648389) -> (12.601873, -6.896998)
  ellipse E616 centre (-9.726318, -5.8407) end of major axis (-8.22635, -5.83093) minor radius 0.235872 (-9.202665, -5.616337) -> (-9.219843, -5.615458) ccw
  ellipse E617 centre (-9.726318, -5.8407) end of major axis (-7.826359, -5.828324) minor radius 0.298772 (-9.19622, -5.550419) -> (-10.866536, -5.608949) ccw
  ellipse E618 centre (-9.744328, -3.075593) end of major axis (-11.644288, -3.087968) minor radius 0.298772 (-11.564332, -3.001391) -> (-11.644288, -3.087968) ccw
  line L751 (-11.634791, -4.546078) -> (-11.644288, -3.087968)
  ellipse E619 centre (7.406411, -6.669461) end of major axis (9.297423, -6.484872) minor radius 0.109208 (9.14693, -6.543029) -> (9.026399, -6.455251) ccw
  ellipse E620 centre (7.134835, -3.887313) end of major axis (9.025847, -3.702725) minor radius 0.109208 (9.025847, -3.702725) -> (8.313284, -3.68685) ccw
  line L752 (9.297423, -6.484872) -> (9.025847, -3.702725)
  ellipse E621 centre (-7.396457, -6.668335) end of major axis (-9.287441, -6.483459) minor radius 0.109208 (-9.016412, -6.453879) -> (-9.136956, -6.541638) ccw
  ellipse E622 centre (-7.124458, -3.886229) end of major axis (-9.015442, -3.701352) minor radius 0.109208 (-8.302877, -3.685586) -> (-9.015442, -3.701352) ccw
  line L753 (-9.287441, -6.483459) -> (-9.015442, -3.701352)
  ellipse E623 centre (9.736398, -5.84218) end of major axis (11.236365, -5.852178) minor radius 0.235872 (9.229957, -5.616861) -> (9.212779, -5.617737) ccw
  ellipse E624 centre (9.736398, -5.84218) end of major axis (11.636356, -5.854844) minor radius 0.298772 (10.876651, -5.610602) -> (9.206344, -5.551818) ccw
  ellipse E625 centre (9.754829, -3.077076) end of major axis (11.654787, -3.08974) minor radius 0.298772 (11.654787, -3.08974) -> (11.574844, -3.003151) ccw
  line L754 (11.645068, -4.547848) -> (11.654787, -3.08974)
  line L755 (-8.740167, -12.052645) -> (-8.723713, -12.15308)
  line L756 (-8.707345, -12.252986) -> (-7.513298, -19.541116)
  line L757 (-3.535044, -19.95765) -> (-2.676231, -17.750224)
  line L758 (-3.535127, -19.957677) -> (-3.535044, -19.95765)
  line L759 (-8.161634, -6.527157) -> (-8.541789, -10.157967)
  line L760 (-8.739665, -12.047845) -> (-8.740167, -12.052645)
  line L761 (-8.161717, -6.527184) -> (-8.23765, -7.25241)
  line L762 (-3.607009, -19.950151) -> (-3.535127, -19.957677)
  line L763 (-7.513298, -19.541116) -> (-7.090722, -19.585361)
  line L764 (-5.432283, -19.759004) -> (-3.535044, -19.95765)
  ellipse E626 centre (-8.161799, -6.527212) end of major axis (-8.214699, -7.03245) minor radius 0.000079 (-8.161717, -6.527184) -> (-8.137299, -6.293894) ccw
  ellipse E627 centre (-8.161799, -6.527212) end of major axis (-8.267599, -7.537688) minor radius 0.000159 (-8.161634, -6.527156) -> (-8.1128, -6.060576) ccw
  ellipse E628 centre (-7.480361, -0.013779) end of major axis (-7.374562, 0.996697) minor radius 0.000159 (-7.431362, 0.452856) -> (-7.374562, 0.996697) ccw
  ellipse E629 centre (-7.480361, -0.013779) end of major axis (-7.427462, 0.491459) minor radius 0.000079 (-7.455862, 0.219538) -> (-7.427462, 0.491459) ccw
  line L765 (-7.374562, 0.996697) -> (-7.064164, 0.964198)
  line L766 (-8.1373, -6.293894) -> (-7.455862, 0.219538)
  line L767 (-8.1128, -6.060577) -> (-7.431362, 0.452856)
  line L768 (-7.374725, 0.996643) -> (-8.369803, 1.100605)
  line L769 (-8.422703, 0.595367) -> (-8.369803, 1.100605)
  line L770 (-8.422703, 0.595367) -> (-7.427625, 0.491405)
  line L771 (-7.374725, 0.996643) -> (-7.427625, 0.491405)
  line L772 (-8.369803, 1.100605) -> (-8.369891, 1.100576)
  line L773 (-7.427625, 0.491405) -> (-7.427462, 0.491459)
  line L774 (-7.374562, 0.996697) -> (-7.374725, 0.996643)
  line L775 (-3.994942, -5.598932) -> (-3.994993, -6.275126)
  line L776 (4.005058, -5.59954) -> (4.005007, -6.275734)
  line L777 (-3.994942, -5.598932) -> (-3.994907, -5.14429)
  line L778 (4.005058, -5.59954) -> (4.005093, -5.144898)
  line L779 (-3.994907, -5.14429) -> (-3.994871, -4.67207)
  line L780 (4.005129, -4.672679) -> (4.005093, -5.144898)
  line L781 (4.327085, 1.254223) -> (4.005588, 1.35998)
  line L782 (4.005549, 0.854739) -> (4.264899, 0.769425)
  line L783 (-3.994412, 1.360588) -> (-4.315926, 1.25488)
  line L784 (-4.253814, 0.770073) -> (-3.994451, 0.855347)
  line L785 (3.542977, -19.958188) -> (3.54306, -19.958215)
  line L786 (2.684499, -17.750632) -> (3.542977, -19.958188)
  line L787 (7.521293, -19.542259) -> (8.716449, -12.254311)
  line L788 (8.732832, -12.154408) -> (8.749302, -12.053975)
  line L789 (8.247515, -7.253663) -> (8.171692, -6.528426)
  line L790 (8.171609, -6.528399) -> (8.551213, -10.159267)
  line L791 (8.7488, -12.049175) -> (8.749302, -12.053975)
  line L792 (3.54306, -19.958215) -> (3.614943, -19.9507)
  line L793 (3.542977, -19.958188) -> (5.440246, -19.75983)
  line L794 (7.098711, -19.58644) -> (7.521293, -19.542259)
  ellipse E630 centre (8.171775, -6.528454) end of major axis (8.118952, -6.023208) minor radius 0.000079 (8.14731, -6.295133) -> (8.171692, -6.528426) ccw
  ellipse E631 centre (8.171775, -6.528454) end of major axis (8.277421, -7.538946) minor radius 0.000159 (8.122846, -6.061811) -> (8.171609, -6.528398) ccw
  ellipse E632 centre (7.491328, -0.014918) end of major axis (7.385682, 0.995575) minor radius 0.000159 (7.385682, 0.995575) -> (7.442399, 0.451725) ccw
  ellipse E633 centre (7.491328, -0.014918) end of major axis (7.438505, 0.490328) minor radius 0.000079 (7.438505, 0.490328) -> (7.466863, 0.218403) ccw
  line L795 (7.075279, 0.963122) -> (7.385682, 0.995575)
  line L796 (8.14731, -6.295133) -> (7.466863, 0.218403)
  line L797 (7.442399, 0.451725) -> (8.122846, -6.061811)
  line L798 (8.380938, 1.099331) -> (7.385845, 0.99552)
  line L799 (7.438667, 0.490274) -> (7.385845, 0.99552)
  line L800 (7.438667, 0.490274) -> (8.433761, 0.594085)
  line L801 (8.433761, 0.594085) -> (8.380938, 1.099331)
  line L802 (8.381027, 1.099302) -> (8.380938, 1.099331)
  line L803 (7.385845, 0.99552) -> (7.385682, 0.995575)
  line L804 (7.438505, 0.490328) -> (7.438667, 0.490274)
  line L805 (-2.977842, -18.525461) -> (-1.996198, -22.119352)
  line L806 (2.003802, -22.119656) -> (2.985992, -18.525914)
  line L807 (-1.996198, -22.119352) -> (2.003802, -22.119656)
  line L808 (-2.371614, -21.797724) -> (-1.996277, -23.162592)
  line L809 (2.003723, -23.162896) -> (2.376691, -21.807448)
  line L810 (-1.996277, -23.162592) -> (2.003723, -23.162896)
  line L811 (-8.363588, -21.430013) -> (-9.500039, -13.927288)
  line L812 (-8.363537, -21.429993) -> (-8.363588, -21.430013)
  line L813 (-9.499988, -13.927269) -> (-8.363537, -21.429993)
  line L814 (-9.500039, -13.927288) -> (-9.499988, -13.927269)
  line L815 (-4.390597, -21.894484) -> (-3.606995, -19.950116)
  line L816 (-4.390649, -21.894504) -> (-4.390597, -21.894484)
  line L817 (-8.854845, -8.40916) -> (-9.499988, -13.927269)
  line L818 (-8.854897, -8.40918) -> (-9.500039, -13.927288)
  line L819 (-8.363588, -21.430013) -> (-4.390649, -21.894504)
  line L820 (-8.363537, -21.429993) -> (-4.390597, -21.894484)
  ellipse E634 centre (-8.854948, -8.4092) end of major axis (-8.913939, -8.913763) minor radius 0.000049 (-8.854897, -8.409179) -> (-8.827664, -8.1762) ccw
  ellipse E635 centre (-8.854948, -8.4092) end of major axis (-8.972929, -9.418327) minor radius 0.000097 (-8.854845, -8.409158) -> (-8.800379, -7.9432) ccw
  ellipse E636 centre (-8.094779, -1.904416) end of major axis (-7.976798, -0.895289) minor radius 0.000097 (-8.04021, -1.438418) -> (-7.976798, -0.895289) ccw
  ellipse E637 centre (-8.094779, -1.904416) end of major axis (-8.035789, -1.399853) minor radius 0.000049 (-8.067495, -1.671417) -> (-8.035789, -1.399853) ccw
  line L821 (-7.976798, -0.895289) -> (-7.577381, -0.941987)
  line L822 (-8.827664, -8.176201) -> (-8.067495, -1.671417)
  line L823 (-8.80038, -7.943202) -> (-8.04021, -1.438418)
  line L824 (-7.976899, -0.895328) -> (-8.970454, -0.779328)
  line L825 (-9.029444, -1.283892) -> (-8.970454, -0.779328)
  line L826 (-9.029444, -1.283892) -> (-8.03589, -1.399891)
  line L827 (-7.976899, -0.895328) -> (-8.03589, -1.399891)
  line L828 (-8.970454, -0.779328) -> (-8.970524, -0.779356)
  line L829 (-8.03589, -1.399891) -> (-8.035789, -1.399853)
  line L830 (-7.976798, -0.895289) -> (-7.976899, -0.895328)
  line L831 (-1.996054, -20.223626) -> (-3.995501, -12.952819)
  line L832 (-1.996049, -20.164739) -> (-1.996054, -20.223626)
  line L833 (-3.995496, -12.893933) -> (-1.996049, -20.164739)
  line L834 (-3.995501, -12.952819) -> (-3.995496, -12.893933)
  line L835 (4.004499, -12.953428) -> (2.003946, -20.22393)
  line L836 (4.004504, -12.894541) -> (4.004499, -12.953428)
  line L837 (2.003951, -20.165043) -> (4.004504, -12.894541)
  line L838 (2.003946, -20.22393) -> (2.003951, -20.165043)
  line L839 (-3.995077, -7.375692) -> (-3.995496, -12.893933)
  line L840 (4.004923, -7.3763) -> (4.004504, -12.894541)
  line L841 (-1.996054, -20.223626) -> (2.003946, -20.22393)
  line L842 (-1.996049, -20.164739) -> (2.003951, -20.165043)
  line L843 (-3.995077, -7.375692) -> (-3.995042, -6.923025)
  line L844 (4.004923, -7.3763) -> (4.004958, -6.923634)
  line L845 (-3.995042, -6.923025) -> (-3.994993, -6.275126)
  line L846 (4.005007, -6.275734) -> (4.004958, -6.923634)
  line L847 (4.218023, -0.568854) -> (4.005447, -0.490969)
  line L848 (4.005408, -0.995544) -> (4.158002, -1.051452)
  line L849 (-3.994553, -0.49036) -> (-4.207141, -0.568213)
  line L850 (-4.147194, -1.050821) -> (-3.994592, -0.994936)
  line L851 (4.398236, -21.895153) -> (4.398287, -21.895173)
  line L852 (3.614929, -19.950665) -> (4.398236, -21.895153)
  line L853 (9.508889, -13.928734) -> (8.371297, -21.431286)
  line L854 (9.508838, -13.928714) -> (9.508889, -13.928734)
  line L855 (8.371246, -21.431266) -> (9.508838, -13.928714)
  line L856 (8.371297, -21.431286) -> (8.371246, -21.431266)
  line L857 (9.508889, -13.928734) -> (8.864586, -8.410528)
  line L858 (8.864535, -8.410508) -> (9.508838, -13.928714)
  line L859 (4.398287, -21.895173) -> (8.371297, -21.431286)
  line L860 (4.398236, -21.895153) -> (8.371246, -21.431266)
  ellipse E638 centre (8.864637, -8.410548) end of major axis (8.805724, -7.905975) minor radius 0.000049 (8.837388, -8.177544) -> (8.864586, -8.410528) ccw
  ellipse E639 centre (8.864637, -8.410548) end of major axis (8.982465, -9.419692) minor radius 0.000097 (8.810139, -7.944539) -> (8.864534, -8.410505) ccw
  ellipse E640 centre (8.105457, -1.905648) end of major axis (7.98763, -0.896503) minor radius 0.000097 (7.98763, -0.896503) -> (8.05096, -1.439642) ccw